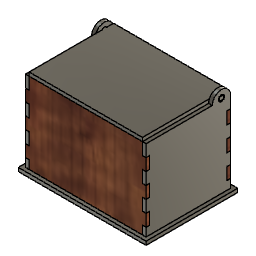
Small Box (Autodesk Fusion 360 design; units mm, degrees)
Autodesk Fusion 360 part; units mm, degrees
sketch "Sketch1" plane through (0, 0, 0) normal (0, 1, 0) x (1, 0, 0) in component "Front"
  line L0 (0, 0) -> (100, 0)
  line L1 (100, 0) -> (100, -70)
  line L2 (100, -70) -> (0, -70)
  line L3 (0, -70) -> (0, 0)
  line L4 (3, -70) -> (3, 0)
  line L5 (0, -10) -> (3, -10)
  line L6 (0, -20) -> (3, -20)
  line L7 (3, -35) -> (3, -30)
  line L8 (3, -30) -> (0, -30)
  line L9 (0, -30) -> (0, -35)
  line L10 (0, -60) -> (3, -60)
  line L11 (3, -60) -> (3, -50)
  line L12 (3, -50) -> (0, -50)
  line L13 (0, -50) -> (0, -60)
  line L14 (0, -40) -> (3, -40)
  line L15 (50, -70) -> (50, 0) construction
  line L16 (100, -60) -> (97, -60)
  line L17 (97, -50) -> (100, -50)
  line L18 (97, -70) -> (97, 0)
  line L19 (100, -40) -> (97, -40)
  line L20 (97, -30) -> (100, -30)
  line L21 (100, -20) -> (97, -20)
  line L22 (100, -10) -> (97, -10)
  line L23 (100, -3) -> (0, -3)
  line L24 (85.7143, -3) -> (71.4286, -3)
  line L25 (71.4286, -3) -> (71.4286, 0)
  line L26 (71.4286, 0) -> (85.7143, 0)
  line L27 (85.7143, 0) -> (85.7143, -3)
  line L28 (57.1429, -3) -> (42.8571, -3)
  line L29 (42.8571, -3) -> (42.8571, 0)
  line L30 (42.8571, 0) -> (57.1429, 0)
  line L31 (57.1429, 0) -> (57.1429, -3)
  line L32 (28.5714, -3) -> (14.2857, -3)
  line L33 (14.2857, -3) -> (14.2857, 0)
  line L34 (14.2857, 0) -> (28.5714, 0)
  line L35 (28.5714, 0) -> (28.5714, -3)
  dimension "d5" = 100
  dimension "d6" = 70
  dimension "d10" = 3
  dimension "d11" = 10
  dimension "d12" = 10
  dimension "d13" = 10
  dimension "d14" = 10
  dimension "d15" = 10
  dimension "d16" = 10
  dimension "d17" = 10
  dimension "d58" = 3
  dimension "d59" = 14.2857
  dimension "d60" = 14.2857
  dimension "d61" = 14.2857
  dimension "d62" = 14.2857
  dimension "d63" = 14.2857
  dimension "d64" = 14.2857
  dimension "d66" = 14.2857
  constraint horizontal L0
  constraint vertical L1
  constraint horizontal L2
  constraint vertical L3
  constraint coincident L0.start L3.end
  constraint coincident L2 L4.start
  constraint coincident L0 L4.end
  constraint perpendicular L0 L4
  constraint coincident L3 L5.start
  constraint coincident L4 L5.end
  constraint perpendicular L4 L5
  constraint coincident L3 L6.start
  constraint coincident L4 L6.end
  constraint perpendicular L4 L6
  constraint vertical L7
  constraint horizontal L8
  constraint vertical L9
  constraint coincident L4 L7.end
  constraint midpoint L3 L9.end
  constraint horizontal L10
  constraint vertical L11
  constraint horizontal L12
  constraint vertical L13
  constraint coincident L4 L11.end
  constraint coincident L3 L10.start
  constraint coincident L3 L14.start
  constraint coincident L4 L14.end
  constraint perpendicular L4 L14
  constraint midpoint L2 L15.start
  constraint midpoint L0 L15.end
  constraint symmetric L4.start L15 L18.start
  constraint symmetric L4.end L15 L18.end
  constraint symmetric L5.start L15 L22.start
  constraint symmetric L5.end L15 L22.end
  constraint symmetric L6.start L15 L21.start
  constraint symmetric L6.end L15 L21.end
  constraint symmetric L7.end L15 L20.start
  constraint symmetric L8.end L15 L20.end
  constraint symmetric L10.start L15 L16.start
  constraint symmetric L10.end L15 L16.end
  constraint symmetric L11.end L15 L17.start
  constraint symmetric L12.end L15 L17.end
  constraint symmetric L14.start L15 L19.start
  constraint symmetric L14.end L15 L19.end
  constraint coincident L1 L23.start
  constraint coincident L3 L23.end
  constraint perpendicular L4 L23
  constraint horizontal L24
  constraint vertical L25
  constraint horizontal L26
  constraint vertical L27
  constraint coincident L0 L25.end
  constraint coincident L23 L24.start
  constraint horizontal L28
  constraint vertical L29
  constraint horizontal L30
  constraint vertical L31
  constraint coincident L23 L28.start
  constraint horizontal L32
  constraint vertical L33
  constraint horizontal L34
  constraint vertical L35
  constraint coincident L0 L33.end
  constraint coincident L23 L32.start
  measures "d5" distance of L0.start L0.end
  measures "d6" distance of L0.end L1.end
  measures "d10" distance of L3 L4
  measures "d11" distance of L5 L6
  measures "d12" distance of L0 L5
  measures "d13" distance of L6 L7.end
  measures "d14" distance of L2 L10
  measures "d15" distance of L10 L12
  measures "d16" distance of L12 L14
  measures "d17" distance of L8 L14
  measures "d58" distance of L0 L23
  measures "d59" distance of L1 L27
  measures "d60" distance of L25 L27
  measures "d61" distance of L25 L31
  measures "d62" distance of L29 L31
  measures "d63" distance of L29 L35
  measures "d64" distance of L33 L35
  measures "d66" distance of L3 L33
extrude "Extrude1" add sketch "Sketch1" against normal blind 3 contours L0 L4 L23 L33 | L2 L4 L7 L11 L18 L23 L24 L28 L32 | L3 L4 L5 L6 | L0 L23 L29 L35 | L3 L4 L7 L8 L9 L14 | L0 L23 L25 L31 | L0 L18 L23 L27 | L3 L4 L10 L11 L12 L13 | L1 L18 L21 L22 | L1 L18 L19 L20 | L1 L16 L17 L18 makes body 1 in component "Front"
sketch "Sketch1 (2)" plane through (0, 0, 0) normal (1, 0, 0) x (0, 1, 0) in component "left"
  line L0 (0, 0) -> (-70, 0)
  line L1 (-70, 0) -> (-70, 70)
  line L2 (-70, 70) -> (0, 70)
  line L3 (0, 70) -> (0, 0)
  line L4 (0, 3) -> (-70, 3)
  line L5 (-10, 3) -> (-20, 3)
  line L6 (-20, 3) -> (-20, 0)
  line L7 (-20, 0) -> (-10, 0)
  line L8 (-10, 0) -> (-10, 3)
  line L9 (-30, 3) -> (-35, 3)
  line L10 (-35, 0) -> (-30, 0)
  line L11 (-30, 0) -> (-30, 3)
  line L12 (-50, 3) -> (-60, 3)
  line L13 (-60, 3) -> (-60, 0)
  line L14 (-60, 0) -> (-50, 0)
  line L15 (-50, 0) -> (-50, 3)
  line L16 (-40, 3) -> (-40, 0)
  circle A0 centre (-7.5677, 70) radius 7.5677
  circle A1 centre (-7.5, 71.5) radius 2.5
  line L17 (-2.98, 70) -> (-2.98, 0)
  line L18 (-2.98, 20) -> (0, 20)
  line L19 (0, 20) -> (0, 10)
  line L20 (0, 10) -> (-2.98, 10)
  line L21 (-2.98, 10) -> (-2.98, 20)
  line L22 (0, 30) -> (-2.98, 30)
  line L23 (-2.98, 30) -> (-2.98, 40)
  line L24 (-2.98, 40) -> (0, 40)
  line L25 (0, 40) -> (0, 30)
  line L26 (-2.98, 50) -> (0, 50)
  line L27 (0, 50) -> (0, 60)
  line L28 (0, 60) -> (-2.98, 60)
  line L29 (-2.98, 60) -> (-2.98, 50)
  line L30 (-35, 70) -> (-35, 0) construction
  line L31 (-67.02, 70) -> (-67.02, 0)
  line L32 (-70, 60) -> (-67.02, 60)
  line L33 (-67.02, 50) -> (-70, 50)
  line L34 (-67.02, 40) -> (-70, 40)
  line L35 (-70, 30) -> (-67.02, 30)
  line L36 (-67.02, 20) -> (-70, 20)
  line L37 (-70, 10) -> (-67.02, 10)
  dimension "d43" = 70
  dimension "d44" = 70
  dimension "d67" = 3
  dimension "d68" = 10
  dimension "d69" = 10
  dimension "d70" = 10
  dimension "d72" = 10
  dimension "d73" = 10
  dimension "d75" = 10
  dimension "d76" = 10
  dimension "d106" = 5
  dimension "d107" = 10
  dimension "d108" = 10
  dimension "d109" = 10
  dimension "d110" = 10
  dimension "d111" = 10
  dimension "d112" = 10
  dimension "d114" = 10
  constraint horizontal L0
  constraint vertical L1
  constraint horizontal L2
  constraint vertical L3
  constraint coincident L0.start L3.end
  constraint coincident L3 L4.start
  constraint coincident L1 L4.end
  constraint perpendicular L1 L4
  constraint horizontal L5
  constraint vertical L6
  constraint horizontal L7
  constraint vertical L8
  constraint coincident L0 L6.end
  constraint coincident L4 L5.start
  constraint horizontal L9
  constraint horizontal L10
  constraint vertical L11
  constraint midpoint L0 L10.start
  constraint coincident L4 L9.start
  constraint horizontal L12
  constraint vertical L13
  constraint horizontal L14
  constraint vertical L15
  constraint coincident L0 L13.end
  constraint coincident L4 L12.start
  constraint coincident L4 L16.start
  constraint coincident L0 L16.end
  constraint perpendicular L0 L16
  constraint coincident L2 A0.centre
  constraint coincident L2.end A0
  constraint coincident L2 L17.start
  constraint coincident L0 L17.end
  constraint perpendicular L0 L17
  constraint horizontal L18
  constraint vertical L19
  constraint horizontal L20
  constraint vertical L21
  constraint coincident L3 L19.end
  constraint coincident L17 L18.start
  constraint horizontal L22
  constraint vertical L23
  constraint horizontal L24
  constraint vertical L25
  constraint coincident L17 L23.end
  constraint coincident L3 L22.start
  constraint horizontal L26
  constraint vertical L27
  constraint horizontal L28
  constraint vertical L29
  constraint coincident L3 L27.end
  constraint coincident L17 L26.start
  constraint midpoint L2 L30.start
  constraint symmetric L17.start L30 L31.start
  constraint symmetric L17.end L30 L31.end
  constraint symmetric L18.start L30 L36.start
  constraint symmetric L18.end L30 L36.end
  constraint symmetric L19.end L30 L37.start
  constraint symmetric L20.end L30 L37.end
  constraint symmetric L22.start L30 L35.start
  constraint symmetric L22.end L30 L35.end
  constraint symmetric L23.end L30 L34.start
  constraint symmetric L24.end L30 L34.end
  constraint symmetric L26.start L30 L33.start
  constraint symmetric L26.end L30 L33.end
  constraint symmetric L27.end L30 L32.start
  constraint symmetric L28.end L30 L32.end
  measures "d43" distance of L1.end L2.end
  measures "d44" distance of L0.end L1.end
  measures "d67" distance of L0 L4
  measures "d68" distance of L3 L8
  measures "d69" distance of L6 L8
  measures "d70" distance of L6 L11
  measures "d72" distance of L1 L13
  measures "d73" distance of L13 L15
  measures "d75" distance of L15 L16
  measures "d76" distance of L11 L16
  measures "d106" diameter of A1
  measures "d107" distance of L26 L28
  measures "d108" distance of L2 L27.end
  measures "d109" distance of L24 L26
  measures "d110" distance of L22.start L24
  measures "d111" distance of L18 L22
  measures "d112" distance of L18 L20
  measures "d114" distance of L0 L20
extrude "Extrude1'" add sketch "Sketch1 (2)" along normal blind 3 separate body contours L3 L4 L17 L20 | L0 L4 L5 L6 L7 L8 | L2 L4 L5 L9 L12 A0 L17 L21 L23 L29 L31 | L3 L17 L18 L22 | L0 L4 L9 L10 L11 L16 | L3 L17 L24 L26 | L0 L4 L12 L13 L14 L15 | L3 A0 L17 L28 | L2 A0 L17 | L2 A0 A1 | L2 A0 A1 L17 | L1 L4 L31 L37 | L1 L2 L31 L32 | L1 L31 L35 L36 | L1 L31 L33 L34 makes body 2 in component "left"
ref_plane "WorkPlane3" through (50, -35, 35) normal (0, 1, 0) x (1, 0, 0)
mirror "Mirror4" about plane through (50, -35, 35) normal (0, 1, 0) of bodies 1 makes body 3 in component "Front"
ref_plane "WorkPlane5" through (50, -35, 38.7839) normal (1, 0, 0) x (0, 1, 0)
mirror "Mirror1" about plane through (50, -35, 38.7839) normal (1, 0, 0) of bodies 2 makes body 4 in component "left"
sketch "Sketch2" plane through (0, 0, 0) normal (0, 0, 1) x (1, 0, 0) in component "base"
  line L0 (0, 0) -> (100, 0)
  line L1 (100, 0) -> (100, -70)
  line L2 (100, -70) -> (0, -70)
  line L3 (0, -70) -> (0, 0)
  line L4 (103, -73) -> (-3, -73)
  line L5 (-3, -73) -> (-3, 3)
  line L6 (-3, 3) -> (103, 3)
  line L7 (103, 3) -> (103, -73)
  dimension "d81" = 100
  dimension "d82" = 70
  constraint horizontal L0
  constraint vertical L1
  constraint horizontal L2
  constraint vertical L3
  constraint coincident L0.start L3.end
  measures "d81" distance of L1.end L2.end
  measures "d82" distance of L0.end L1.end
extrude "Extrude1''" add sketch "Sketch2" along normal blind 3 separate body contours L0 L1 L2 L3 | L4 L5 L6 L7 makes body 5 in component "base"
combine "Combine1" operation cut target body 5 tool bodies 4 1 3 2 keep tools in component "base"
sketch "Sketch1 (3)" plane through (0, 0, 0) normal (0, 0, 1) x (1, 0, 0) in component "lid"
  line L0 (0, 0) -> (100, 0)
  line L1 (100, 0) -> (100, -70)
  line L2 (100, -70) -> (0, -70)
  line L3 (0, -70) -> (0, 0)
  line L4 (3, 0) -> (3, -70)
  line L5 (0, -6) -> (3, -6)
  line L6 (3, -6) -> (3, -9)
  line L7 (3, -9) -> (0, -9)
  line L8 (0, -9) -> (0, -6)
  line L9 (50, 0) -> (50, -70) construction
  line L10 (97, 0) -> (97, -70)
  line L11 (100, -6) -> (97, -6)
  line L12 (97, -9) -> (100, -9)
  line L13 (0, -67) -> (100, -67)
  dimension "d98" = 3
  dimension "d99" = 3
  dimension "d100" = 6
  dimension "d103" = 3
  constraint horizontal L0
  constraint vertical L1
  constraint horizontal L2
  constraint vertical L3
  constraint coincident L0.start L3.end
  constraint coincident L0 L4.start
  constraint coincident L2 L4.end
  constraint perpendicular L2 L4
  constraint horizontal L5
  constraint vertical L6
  constraint horizontal L7
  constraint vertical L8
  constraint coincident L4 L6.end
  constraint coincident L3 L5.start
  constraint midpoint L0 L9.start
  constraint midpoint L2 L9.end
  constraint symmetric L4.start L9 L10.start
  constraint symmetric L4.end L9 L10.end
  constraint symmetric L5.start L9 L11.start
  constraint symmetric L5.end L9 L11.end
  constraint symmetric L6.end L9 L12.start
  constraint symmetric L7.end L9 L12.end
  constraint coincident L3 L13.start
  constraint coincident L1 L13.end
  constraint perpendicular L1 L13
  measures "d98" distance of L5 L7
  measures "d99" distance of L3 L4
  measures "d100" distance of L0 L5
  measures "d103" distance of L2 L13
extrude "Extrude1'''" add sketch "Sketch1 (3)" along normal blind 3 separate body contours L0 L4 L6 L10 L13 | L3 L4 L5 L6 L7 L8 | L1 L10 L11 L12 | L2 L4 L10 L13 makes body 6 in component "lid"
sketch "Front_DXF" plane through (0, -70, 0) normal (0, -1, 0) x (1, 0, 0)
  line L0 (57.1429, 3) -> (57.1429, 0)
  line L1 (57.1429, 0) -> (71.4286, 0)
  line L2 (71.4286, 0) -> (71.4286, 3)
  line L3 (71.4286, 3) -> (85.7143, 3)
  line L4 (85.7143, 3) -> (85.7143, 0)
  line L5 (85.7143, 0) -> (97, 0)
  line L6 (97, 0) -> (97, 10)
  line L7 (97, 10) -> (100, 10)
  line L8 (100, 10) -> (100, 20)
  line L9 (100, 20) -> (97, 20)
  line L10 (97, 20) -> (97, 30)
  line L11 (97, 30) -> (100, 30)
  line L12 (100, 30) -> (100, 40)
  line L13 (100, 40) -> (97, 40)
  line L14 (97, 40) -> (97, 50)
  line L15 (97, 50) -> (100, 50)
  line L16 (100, 50) -> (100, 60)
  line L17 (100, 60) -> (97, 60)
  line L18 (97, 60) -> (97, 70)
  line L19 (97, 70) -> (3, 70)
  line L20 (3, 70) -> (3, 60)
  line L21 (3, 60) -> (0, 60)
  line L22 (0, 60) -> (0, 50)
  line L23 (0, 50) -> (3, 50)
  line L24 (3, 50) -> (3, 40)
  line L25 (3, 40) -> (0, 40)
  line L26 (0, 40) -> (0, 30)
  line L27 (0, 30) -> (3, 30)
  line L28 (3, 30) -> (3, 20)
  line L29 (3, 20) -> (0, 20)
  line L30 (0, 20) -> (0, 10)
  line L31 (0, 10) -> (3, 10)
  line L32 (3, 10) -> (3, 0)
  line L33 (3, 0) -> (14.2857, 0)
  line L34 (14.2857, 0) -> (14.2857, 3)
  line L35 (14.2857, 3) -> (28.5714, 3)
  line L36 (28.5714, 3) -> (28.5714, 0)
  line L37 (28.5714, 0) -> (42.8571, 0)
  line L38 (42.8571, 0) -> (42.8571, 3)
  line L39 (42.8571, 3) -> (57.1429, 3)
sketch "Base_DXF" plane through (0, 0, 3) normal (0, 0, 1) x (-1, 0, 0)
  line L0 (-3, 0) -> (-14.2857, 0)
  line L1 (-14.2857, 0) -> (-14.2857, 3)
  line L2 (-14.2857, 3) -> (-3, 3)
  line L3 (-3, 3) -> (-3, 0)
  line L4 (0, 10) -> (-3, 10)
  line L5 (-3, 20) -> (0, 20)
  line L6 (0, 20) -> (0, 10)
  line L7 (0, 30) -> (-3, 30)
  line L8 (-3, 40) -> (0, 40)
  line L9 (0, 40) -> (0, 30)
  line L10 (-3, 67) -> (-14.2857, 67)
  line L11 (-14.2857, 67) -> (-14.2857, 70)
  line L12 (-14.2857, 70) -> (-3, 70)
  line L13 (-3, 70) -> (-3, 67)
  line L14 (-103, -3) -> (3, -3)
  line L15 (3, -3) -> (3, 73)
  line L16 (3, 73) -> (-103, 73)
  line L17 (-103, 73) -> (-103, -3)
  line L18 (-100, 60) -> (-97, 60)
  line L19 (-71.4286, 0) -> (-71.4286, 3)
  line L20 (-71.4286, 3) -> (-57.1429, 3)
  line L21 (-57.1429, 3) -> (-57.1429, 0)
  line L22 (-57.1429, 0) -> (-71.4286, 0)
  line L23 (-28.5714, 3) -> (-28.5714, 0)
  line L24 (-28.5714, 0) -> (-42.8571, 0)
  line L25 (-42.8571, 0) -> (-42.8571, 3)
  line L26 (-42.8571, 3) -> (-28.5714, 3)
  line L27 (-85.7143, 0) -> (-97, 0)
  line L28 (-97, 0) -> (-97, 3)
  line L29 (-97, 3) -> (-85.7143, 3)
  line L30 (-85.7143, 3) -> (-85.7143, 0)
  line L31 (-71.4286, 67) -> (-71.4286, 70)
  line L32 (-71.4286, 70) -> (-57.1429, 70)
  line L33 (-57.1429, 70) -> (-57.1429, 67)
  line L34 (-57.1429, 67) -> (-71.4286, 67)
  line L35 (-28.5714, 70) -> (-28.5714, 67)
  line L36 (-28.5714, 67) -> (-42.8571, 67)
  line L37 (-42.8571, 67) -> (-42.8571, 70)
  line L38 (-42.8571, 70) -> (-28.5714, 70)
  line L39 (-85.7143, 67) -> (-97, 67)
  line L40 (-97, 67) -> (-97, 70)
  line L41 (-97, 70) -> (-85.7143, 70)
  line L42 (-85.7143, 70) -> (-85.7143, 67)
  line L43 (0, 50) -> (-3, 50)
  line L44 (0, 60) -> (0, 50)
  line L45 (-3, 10) -> (-3, 20)
  line L46 (-3, 30) -> (-3, 40)
  line L47 (-97, 50) -> (-100, 50)
  line L48 (-100, 50) -> (-100, 60)
  line L49 (-97, 60) -> (-97, 50)
  line L50 (-97, 30) -> (-100, 30)
  line L51 (-100, 30) -> (-100, 40)
  line L52 (-100, 40) -> (-97, 40)
  line L53 (-97, 40) -> (-97, 30)
  line L54 (-97, 10) -> (-100, 10)
  line L55 (-100, 10) -> (-100, 20)
  line L56 (-100, 20) -> (-97, 20)
  line L57 (-97, 20) -> (-97, 10)
  line L58 (-3, 50) -> (-3, 60)
  line L59 (-3, 60) -> (0, 60)
move_body "Move2" bodies 6 to x (1, 0, 0) y (0, 1, 0) z (0, 0, 1) at (0, 0, 70) in component "lid"
sketch "Lid_DXF" plane through (0, 0, 73) normal (0, 0, 1) x (-1, 0, 0)
  line L0 (-97, 70) -> (-97, 9)
  line L1 (-97, 9) -> (-100, 9)
  line L2 (-100, 9) -> (-100, 6)
  line L3 (-100, 6) -> (-97, 6)
  line L4 (-97, 6) -> (-97, 0)
  line L5 (-97, 0) -> (-3, 0)
  line L6 (-3, 0) -> (-3, 6)
  line L7 (-3, 6) -> (0, 6)
  line L8 (0, 6) -> (0, 9)
  line L9 (0, 9) -> (-3, 9)
  line L10 (-3, 9) -> (-3, 70)
  line L11 (-3, 70) -> (-97, 70)
sketch "Left_DXF" plane through (100, 0, 0) normal (1, 0, 0) x (0, 1, 0)
  circle A0 centre (-7.5, 71.5) radius 2.5
  line L0 (-60, 3) -> (-60, 0)
  line L1 (-60, 0) -> (-50, 0)
  line L2 (-50, 0) -> (-50, 3)
  line L3 (-50, 3) -> (-40, 3)
  line L4 (-40, 3) -> (-40, 0)
  line L5 (-40, 0) -> (-30, 0)
  line L6 (-30, 0) -> (-30, 3)
  line L7 (-30, 3) -> (-20, 3)
  line L8 (-20, 3) -> (-20, 0)
  line L9 (-20, 0) -> (-10, 0)
  line L10 (-10, 0) -> (-10, 3)
  line L11 (-10, 3) -> (0, 3)
  line L12 (0, 3) -> (0, 10)
  line L13 (0, 10) -> (-2.98, 10)
  line L14 (-2.98, 10) -> (-2.98, 20)
  line L15 (-2.98, 20) -> (0, 20)
  line L16 (0, 20) -> (0, 30)
  line L17 (0, 30) -> (-2.98, 30)
  line L18 (-2.98, 30) -> (-2.98, 40)
  line L19 (-2.98, 40) -> (0, 40)
  line L20 (0, 40) -> (0, 50)
  line L21 (0, 50) -> (-2.98, 50)
  line L22 (-2.98, 50) -> (-2.98, 60)
  line L23 (-2.98, 60) -> (0, 60)
  line L24 (0, 60) -> (0, 70)
  arc A1 (0, 70) -> (-15.1355, 70) centre (-7.5677, 70) ccw
  line L25 (-15.1355, 70) -> (-70, 70)
  line L26 (-70, 70) -> (-70, 60)
  line L27 (-70, 60) -> (-67.02, 60)
  line L28 (-67.02, 60) -> (-67.02, 50)
  line L29 (-67.02, 50) -> (-70, 50)
  line L30 (-70, 50) -> (-70, 40)
  line L31 (-70, 40) -> (-67.02, 40)
  line L32 (-67.02, 40) -> (-67.02, 30)
  line L33 (-67.02, 30) -> (-70, 30)
  line L34 (-70, 30) -> (-70, 20)
  line L35 (-70, 20) -> (-67.02, 20)
  line L36 (-67.02, 20) -> (-67.02, 10)
  line L37 (-67.02, 10) -> (-70, 10)
  line L38 (-70, 10) -> (-70, 3)
  line L39 (-70, 3) -> (-60, 3)
component "Front" placed x (1, 0, 0) y (0, 1, 0) z (0, 0, 1) at (0, 0, 0)
component "left" placed x (1, 0, 0) y (0, 1, 0) z (0, 0, 1) at (0, 0, 0)
component "base" placed x (1, 0, 0) y (0, 1, 0) z (0, 0, 1) at (0, 0, 0)
component "lid" placed x (1, 0, 0) y (0, 1, 0) z (0, 0, 1) at (0, 0, 0)
equation "length = 100 mm"
equation "width = 70 mm"
equation "height = 70 mm"
equation "thickness = 3 mm"
equation "d5 = length"
equation "d6 = height"
equation "lfinger = 3" comment "number of fingers for length"
equation "hfinger = 3" comment "number of fingers for height"
equation "wfinger = 3" comment "number of fingers for width"
equation "d10 = thickness"
equation "d11 = height / ( 2 * hfinger + 1 )"
equation "d12 = d11"
equation "d13 = d11"
equation "d14 = d13"
equation "d15 = d14"
equation "d16 = d15"
equation "d18 = -thickness"
equation "d24 = height / ( 2 * hfinger + 1 )"
equation "d25 = d24"
equation "d26 = d25"
equation "d27 = d26"
equation "d28 = d27"
equation "d43 = width"
equation "d44 = height"
equation "d45 = thickness"
equation "d58 = thickness"
equation "d59 = ( length / ( ( lfinger * 2 ) * 1 mm + 1 mm ) ) * 1 mm"
equation "d60 = d59"
equation "d61 = d60"
equation "d62 = d61"
equation "d63 = d61"
equation "d64 = d63"
equation "d67 = thickness"
equation "d68 = width / ( wfinger * 2 + 1 )"
equation "d69 = d68"
equation "d70 = d69"
equation "d72 = d70"
equation "d73 = d72"
equation "d75 = d73"
equation "d81 = length"
equation "d82 = width"
equation "d83 = -thickness"
equation "d84 = thickness"
equation "d98 = thickness"
equation "d99 = thickness"
equation "d101 = thickness"
equation "d103 = thickness"
equation "d107 = height / ( hfinger * 2 + 1 )"
equation "d108 = d107"
equation "d109 = d107"
equation "d110 = d109"
equation "d111 = d110"
equation "d112 = d111"
